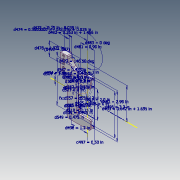
# Autodesk Inventor part: J005316
Saved by Autodesk Inventor 2015 SP1 (Build 190203100, 203)
## iProperties
Created: 2014-10-30
Material: ALUMINUM, 6061-T651
Vendor: HHMI: JRC - ID&F
Document SubType Name: Modeling
Designer: arnoldj
Density: 2.7 g/cm^3
Mass: 47.9365 g
Surface Area: 89.1048 cm^2
Volume: 17.7543 cm^3
Description: MBS INLINE CLAMP ARM
Project: P-201804
Appearance: Metal-AL-6061 (Machined)
Part Number: J005316
RuleStatus: InUse
AfterDocSave0: file://Part Number Cleaner
LAB/DEPT: SVOBODA (LAB)
REQUESTING SCIENTIST: SOFRONIEW, NICK
SURFACE ROUGHNESS: 63 Ra
DESIGN DEPARTMENT: HHMI: JRC - ID&F
SPECIAL FINISH: NONE
ALTERED ITEM PART NUMBER: N/A
ALTERED ITEM VENDOR: N/A
ALTERED ITEM DESCRIPTION: N/A
Revision Number: -
Autodesk Inventor part; units mm, degrees
ref_plane "YZ Plane" through (0, 0, 0) normal (1, 0, 0) x (0, 1, 0)
ref_plane "Work Plane13" through (0, 0, -3.81) normal (0, 0, -1) x (-1, 0, 0)
ref_plane "Work Plane14" through (0, 0, -6.35) normal (0, 0, -1) x (-1, 0, 0)
sketch "Sketch1" plane through (0, 0, 0) normal (0, 0, 1) x (1, 0, 0)
  line L0 (0, 79.6138) -> (0, -62.164) projected
  line L1 (-30.389, 41.91) -> (-18.3199, 23.6756)
  line L2 (-29.3116, 41.91) -> (-29.3116, 59.3598)
  line L3 (-34.671, 59.3598) -> (-34.671, 19.4629) construction
  line L4 (-43.9166, 33.4315) -> (-43.9166, 59.3598)
  line L5 (-29.3116, 59.3598) -> (-43.9166, 59.3598)
  line L6 (-30.48, 13.131) -> (-43.9166, 33.4315)
  line L7 (-31.6288, 14.8666) -> (-18.3199, 23.6756)
  line L8 (-69.5376, 0) -> (93.7539, 0) projected
  line L9 (12.573, 37.973) -> (12.573, -37.973) construction
  line L10 (12.573, -37.973) -> (-12.573, -37.973) construction
  line L11 (-12.573, -37.973) -> (-12.573, 37.973) construction
  line L12 (-12.573, 37.973) -> (12.573, 37.973) construction
  line L13 (12.573, 37.973) -> (-12.573, -37.973) construction
  line L14 (12.573, -37.973) -> (-12.573, 37.973) construction
  line L15 (12.7, 41.91) -> (-29.3116, 41.91)
  line L16 (12.7, -41.91) -> (-30.48, -41.91)
  line L17 (-30.48, -41.91) -> (-30.48, 13.131)
  line L18 (12.7, -41.91) -> (12.7, 41.91)
  line L19 (0, 0) -> (70.4266, 0)
  dimension "d473" = 146.5
  dimension "d474" = 9.2456
  dimension "d475" = 5.3594
  dimension "d478" = 25.9283
  dimension "d481" = 25.146
  dimension "d482" = 75.946
  dimension "d483" = 0
  dimension "d492" = 43.9166
  dimension "d493" = 59.3598
  dimension "d494" = 0
  dimension "d495" = 0
  dimension "d496" = 83.82
  dimension "d497" = 12.7
  dimension "d498" = 30.48
  dimension "d499" = 17.4498
  constraints: 36 end point, 5 parallel, 5 point on line, 3 perpendicular, 2 horizontal, 2 midpoint, 2 vertical, 1 other
  measures "d473" angle of L2 L1
  measures "d474" distance between parallel lines of L3 L4
  measures "d475" distance between parallel lines of L3 L2
  measures "d478" distance of L4.start L5.end
  measures "d481" distance of L11.end L9.start
  measures "d482" distance of L10.end L11.end
  measures "d483" angle of L0 L9
  measures "d492" distance from line of L19.start L4
  measures "d493" distance from line of L19.start L5
  measures "d494" distance of L19.start point (0, 0)
  measures "d495" distance of L19.start point (0, 0)
  measures "d496" distance of L16.start L15.start
  measures "d497" distance between parallel lines of L18 L0
  measures "d498" distance between parallel lines of L17 L0
  measures "d499" distance of L2.start L5.start
extrude "Extrusion1" add sketch "Sketch1" along normal blind 7.62
sketch "Sketch32" plane through (0, 0, 0) normal (0, 0, -1) x (-1, 0, 0)
  line L0 (0, -62.164) -> (0, 79.6138) projected
  line L1 (-24.482, 0) -> (57.9922, 0) projected
  point P0 (0, 0)
sketch "Sketch37" plane through (0, 0, 0) normal (0, 0, -1) x (-1, 0, 0)
  line L0 (41.3766, 59.3598) -> (33.1216, 59.3598)
  line L1 (33.1216, 59.3598) -> (41.3766, 59.3598)
  line L2 (41.3766, 59.3598) -> (41.3766, 29.5939)
  line L3 (33.1216, 17.122) -> (41.3766, 29.5939)
  line L4 (33.1216, 17.122) -> (33.1216, 59.3598)
  line L5 (41.3766, 59.3598) -> (33.1216, 59.3598)
  line L6 (43.9166, 59.3598) -> (29.3116, 59.3598) projected
  line L7 (43.9166, 33.4315) -> (43.9166, 59.3598) projected
  line L8 (29.3116, 59.3598) -> (29.3116, 41.91) projected
  line L9 (30.48, 13.131) -> (43.9166, 33.4315) projected
  point P0 (0, 0)
  point P1 (32.8891, 16.7708)
  point P2 (29.3116, 44.1198)
  point P3 (31.6288, 14.8666)
  dimension "d420" = 8.255
  dimension "d560" = 0
  dimension "d561" = 2.54
  constraints: 12 end point, 2 perpendicular, 2 point on line, 8 other
  measures "d420" distance between parallel lines of L2 L4
  measures "d560" distance between parallel lines of L6 L0
  measures "d561" distance between parallel lines of L2 L7
extrude "Extrusion29" add sketch "Sketch37" along normal blind 2.54 contours L2 L3 L4 L0
sketch "Sketch38" plane through (0, 0, -6.35) normal (0, 0, -1) x (-1, 0, 0)
  line L0 (37.2491, 59.3598) -> (37.2491, 23.358) construction
  line L1 (37.2491, 30.3483) -> (43.9166, 30.3483) construction
  line L2 (37.2491, 49.3983) -> (43.9166, 49.3983) construction
  line L3 (37.2491, 43.0483) -> (43.9166, 43.0483) construction
  line L4 (37.2491, 36.6983) -> (43.9166, 36.6983) construction
  circle A0 centre (37.2491, 49.3983) radius 2.5 construction
  circle A1 centre (37.2491, 30.3483) radius 2.5 construction
  line L5 (37.2491, 51.8983) -> (35.7538, 51.8983) construction
  line L6 (37.2491, 55.7483) -> (43.9166, 55.7483) construction
  line L7 (43.9166, 33.4315) -> (43.9166, 59.3598) projected
  line L8 (43.9166, 59.3598) -> (29.3116, 59.3598) projected
  point P0 (41.3766, 59.3598)
  dimension "d415" = 5
  dimension "d407" = 6.35
  dimension "d410" = 6.35
  dimension "d411" = 6.35
  dimension "d412" = 9.9615
  dimension "d413" = 6.9903
  dimension "d416" = 5
  dimension "d427" = 6.35
  dimension "d461" = 19.6903
  dimension "d479" = 6.6675
  dimension "d480" = 9.9615
  constraints: 14 end point, 6 point on line, 2 coincident, 1 centre point, 1 horizontal, 1 parallel, 1 perpendicular, 1 vertical alignment, 2 other
  measures "d407" distance between parallel lines of L2 L3
  measures "d410" distance between parallel lines of L3 L4
  measures "d411" distance between parallel lines of L1 L4
  measures "d412" distance from line of L0.start L2
  measures "d413" distance from line of L0.end L1
  measures "d416" diameter of A1
  measures "d427" distance from line of L2 L6.start
  measures "d461" distance from line of L0.end L3
  measures "d479" distance between parallel lines of L7 L0
  measures "d480" distance from line of L2.start L8
hole "Hole3" at (-37.2491, 43.0483, -6.35) at (-37.2491, 36.6983, -6.35) at (-37.2491, 49.3983, -6.35) at (-37.2491, 55.7483, -6.35) at (-37.2491, 30.3483, -6.35) direction (0, 0, 1) diameter 4.1402 end through all
sketch "Sketch45" plane through (0, 0, 0) normal (0, 0, -1) x (-1, 0, 0)
  line L0 (-12.7, 41.91) -> (-12.7, -41.91) projected
  line L1 (12.7, -38.735) -> (-12.7, -38.735)
  line L2 (-12.7, -38.735) -> (-12.7, 38.735)
  line L3 (-12.7, 38.735) -> (12.7, 38.735)
  line L4 (12.7, 38.735) -> (12.7, -38.735)
  line L5 (12.7, -38.735) -> (-12.7, 38.735) construction
  line L6 (-12.7, -38.735) -> (12.7, 38.735) construction
  line L7 (12.7, 38.735) -> (16.51, 38.735)
  line L8 (16.51, 38.735) -> (16.51, 26.67)
  line L9 (16.51, 26.67) -> (12.7, 26.67)
  line L10 (12.7, 26.67) -> (12.7, 38.735)
  line L11 (12.7, -38.735) -> (16.51, -38.735)
  line L12 (16.51, -38.735) -> (16.51, -26.67)
  line L13 (16.51, -26.67) -> (12.7, -26.67)
  line L14 (12.7, -26.67) -> (12.7, -38.735)
  line L15 (-12.7, 41.91) -> (-12.7, -41.91) projected
  line L16 (12.7, -25.4) -> (-12.7, -25.4)
  line L17 (-12.7, -25.4) -> (-12.7, 25.4)
  line L18 (-12.7, 25.4) -> (12.7, 25.4)
  line L19 (12.7, 25.4) -> (12.7, -25.4)
  line L20 (12.7, -25.4) -> (-12.7, 25.4) construction
  line L21 (-12.7, -25.4) -> (12.7, 25.4) construction
  point P0 (0, 0)
  point P1 (0, 0)
  point P2 (0, 0)
  dimension "d504" = 77.47
  dimension "d505" = 0
  dimension "d506" = 25.4
  dimension "d509" = 12.065
  dimension "d510" = 3.81
  dimension "d511" = 12.065
  dimension "d512" = 3.81
  dimension "d517" = 50.8
  dimension "d519" = 0
  dimension "d521" = 0
  constraints: 40 end point, 8 parallel, 4 horizontal, 4 midpoint, 4 perpendicular, 2 point on line
  measures "d504" distance of L3.end L1.start
  measures "d505" distance of point (0, 0) point (0, 0)
  measures "d506" distance of L2.end L3.end
  measures "d509" distance of L11.end L12.end
  measures "d510" distance of L12.end L13.end
  measures "d511" distance of L7.end L8.end
  measures "d512" distance of L8.end L9.end
  measures "d517" distance of L18.end L16.start
  measures "d519" distance between parallel lines of L4 L19
  measures "d521" distance of point (0, 0) point (0, 0)
extrude "Extrusion33" cut sketch "Sketch45" against normal blind 4.826
extrude "Extrusion34" cut sketch "Sketch45" against normal up to next contours L18 L4 L16 L0
sketch "Sketch46" plane through (0, 0, 0) normal (0, 0, -1) x (-1, 0, 0)
  line L0 (29.3116, 41.91) -> (-12.7, 41.91) projected
  point P0 (0, 0)
sketch "Sketch47" plane through (0, 0, 0) normal (0, 0, -1) x (-1, 0, 0)
  line L0 (29.3116, 41.91) -> (-12.7, 41.91) projected
  line L1 (-12.7, 38.735) -> (16.51, 38.735) projected
  line L2 (-3.175, 41.91) -> (3.175, 41.91)
  line L3 (3.175, 41.91) -> (3.175, 38.735)
  line L4 (3.175, 38.735) -> (-3.175, 38.735)
  line L5 (-3.175, 38.735) -> (-3.175, 41.91)
  line L6 (-12.7, -41.91) -> (30.48, -41.91) projected
  line L7 (16.51, -38.735) -> (-12.7, -38.735) projected
  line L8 (-3.175, -41.91) -> (3.175, -41.91)
  line L9 (3.175, -41.91) -> (3.175, -38.735)
  line L10 (3.175, -38.735) -> (-3.175, -38.735)
  line L11 (-3.175, -38.735) -> (-3.175, -41.91)
  line L12 (0, -41.91) -> (0, -38.735) construction
  line L13 (0, 41.91) -> (0, 38.735) construction
  line L14 (12.7, 26.67) -> (12.7, -26.67) construction
  point P0 (0, 0)
  dimension "d529" = 6.35
  dimension "d530" = 6.35
  dimension "d531" = 12.7
  dimension "d532" = 12.7
  constraints: 20 end point, 4 midpoint, 4 parallel, 4 point on line, 2 horizontal, 2 perpendicular
  measures "d529" distance of L2.start L2.end
  measures "d530" distance of L8.start L8.end
  measures "d531" distance between parallel lines of L14 L12
  measures "d532" distance between parallel lines of L14 L13
extrude "Extrusion35" cut sketch "Sketch47" against normal up to surface (4.826 mm away)
sketch "Sketch50" plane through (0, 0, 0) normal (0, 0, 1) x (1, 0, 0)
  line L0 (-12.7, 26.67) -> (-12.7, 38.735) projected
  line L1 (-12.7, 38.735) -> (-27.94, 38.735)
  line L2 (-27.94, 38.735) -> (-27.94, 26.67)
  line L3 (-27.94, 26.67) -> (-12.7, 26.67)
  line L4 (-12.7, 26.67) -> (-12.7, 38.735)
  line L5 (-12.7, -26.67) -> (-12.7, -38.735) projected
  line L6 (-12.7, -38.735) -> (-27.94, -38.735)
  line L7 (-27.94, -38.735) -> (-27.94, -26.67)
  line L8 (-27.94, -26.67) -> (-12.7, -26.67)
  line L9 (-12.7, -26.67) -> (-12.7, -38.735)
  line L10 (-12.7, -25.4) -> (-12.7, 25.4) projected
  line L11 (-12.7, 22.225) -> (-17.3698, 22.225)
  line L12 (-17.3698, 22.225) -> (-17.3698, -22.225)
  line L13 (-17.3698, -22.225) -> (-12.7, -22.225)
  line L14 (-12.7, -22.225) -> (-12.7, 22.225)
  line L15 (-12.7, 22.225) -> (-17.3698, 17.145)
  line L16 (-12.7, -22.225) -> (-17.3698, -17.145)
  line L17 (-16.51, 38.735) -> (-16.51, 26.67) projected
  point P0 (0, 0)
  dimension "d547" = 12.065
  dimension "d548" = 15.24
  dimension "d549" = 12.065
  dimension "d550" = 15.24
  dimension "d554" = 5.08
  dimension "d555" = 5.08
  dimension "d556" = 44.45
  dimension "d557" = 22.225
  dimension "d562" = 0.8598
  constraints: 28 end point, 6 parallel, 3 horizontal, 3 perpendicular, 3 point on line
  measures "d547" distance of L1.end L2.end
  measures "d548" distance of L2.end L3.end
  measures "d549" distance of L6.end L7.end
  measures "d550" distance of L7.end L8.end
  measures "d554" distance from line of L11 L15.end
  measures "d555" distance from line of L13 L16.end
  measures "d556" distance of L11.end L12.end
  measures "d557" distance from line of point (0, 0) L13
  measures "d562" distance between parallel lines of L17 L12
extrude "Extrusion36" cut sketch "Sketch50" along normal blind 2.54 contours L3 L17 L1 L0 | L3 L2 L1 L17 | L5 L6 L7 L8
extrude "Extrusion37" cut sketch "Sketch50" along normal up to surface (4.826 mm away) contours L16 L12 L15 L10
sketch "Sketch49" plane through (0, 0, 0) normal (0, 0, 1) x (1, 0, 0)
  line L0 (-22.86, 32.004) -> (-22.86, -32.004) construction
  line L1 (0, 79.6138) -> (0, -62.164) projected
  point P0 (0, 0)
  dimension "d537" = 64.008
  dimension "d538" = 32.004
  dimension "d539" = 22.86
  constraints: 2 coincident, 2 end point, 1 vertical
  measures "d537" distance of L0.start L0.end
  measures "d538" vertical distance of L0.end point (0, 0)
  measures "d539" distance between parallel lines of L1 L0
hole "Hole6" at (-22.86, 32.004, 0) at (-22.86, -32.004, 0) at (-22.86, -32.004, 0) direction (0, 0, 1) diameter 2.159 end through all
fillet "Fillet51" radius 1.651 18 edges at (-16.51, 38.735, 3.683) (-16.51, 26.67, 3.683) (-16.51, -26.67, 3.683) (-16.51, -38.735, 3.683) (-12.7, 26.67, 2.413) (-12.7, -26.67, 2.413) (12.7, -25.4, 6.223) (12.7, 25.4, 6.223) (-12.7, 25.4, 6.223) (-12.7, -25.4, 6.223) (-27.94, 38.735, 1.27) (-27.94, 26.67, 1.27) (-27.94, -38.735, 1.27) (-27.94, -26.67, 1.27) (-12.7, 22.225, 2.413) (-17.3698, 17.145, 2.413) (-17.3698, -17.145, 2.413) (-12.7, -22.225, 2.413)
chamfer "Chamfer27" distance 9.525 angle 45 1 edges at (-29.3116, 41.91, 3.81)
fillet "Fillet50" radius 6.604 2 edges at (-29.3116, 51.435, 3.81) (-19.7866, 41.91, 3.81)
fillet "Fillet52" radius 6.604 2 edges at (-30.48, 13.131, 3.81) (-43.9166, 33.4315, 3.81)
chamfer "Chamfer29" distance 1.27 angle 45 10 edges at (7.9375, 38.735, 0) (-14.732, 38.735, 0) (-20.32, 26.67, 0) (-13.1836, 26.1864, 0) (-12.7, 23.9438, 0) (-12.7, -23.9438, 0) (-13.1836, -26.1864, 0) (-20.32, -26.67, 0) (-14.732, -38.735, 0) (7.9375, -38.735, 0)
fillet "Fillet53" radius 1.651 8 edges at (12.7, 41.91, 3.81) (12.7, -41.91, 3.81) (-29.3116, 59.3598, 3.81) (-43.9166, 59.3598, 3.81) (-33.1216, 59.3598, -1.27) (-33.1216, 17.122, -1.27) (-41.3766, 29.5939, -1.27) (-41.3766, 59.3598, -1.27)
fillet "Fillet54" radius 0.635 8 edges at (-3.175, 38.735, 3.048) (-3.175, 41.91, 2.413) (3.175, 38.735, 3.048) (3.175, 41.91, 2.413) (-3.175, -38.735, 3.048) (-3.175, -41.91, 2.413) (3.175, -41.91, 2.413) (3.175, -38.735, 3.048)
fillet "Fillet55" radius 3.302 1 edges at (-30.48, -41.91, 3.81)
sketch "Sketch48" plane through (0, 0, 0) normal (0, 0, 1) x (1, 0, 0)
  circle A0 centre (-20.8102, 26.2497) radius 25.4 construction
  point P0 (0, 0)
  dimension "d536" = 50.8
  constraints: 1 centre point
  measures "d536" diameter of A0
body "Solid1"
